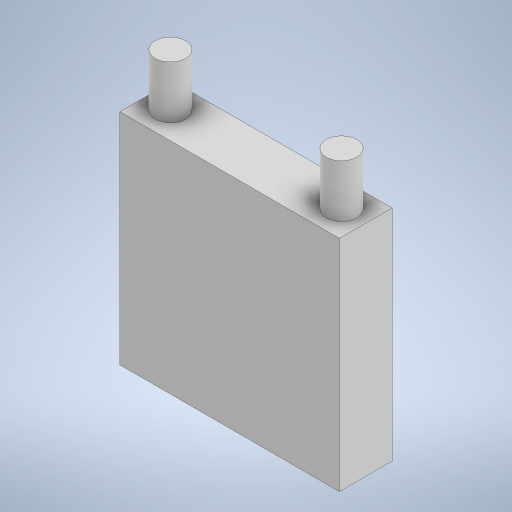
# Autodesk Inventor part: watercoolerpatch
Saved by Autodesk Inventor 2023 (Build 270158000, 158)
## iProperties
Created: 2023-06-13
Part Number: watercoolerpatch
Material: 一般
Document SubType Name: Modeling
Designer: 310611102
Density: 1 g/cm^3
Appearance: 預設
Author: 310611102
Autodesk Inventor part; units mm, degrees
ref_plane "YZ Plane" through (0, 0, 0) normal (1, 0, 0) x (0, 1, 0)
ref_plane "XZ Plane" through (0, 0, 0) normal (0, 1, 0) x (-1, 0, 0)
ref_plane "XY Plane" through (0, 0, 0) normal (0, 0, 1) x (1, 0, 0)
sketch "Sketch1" plane through (0, 0, 0) normal (0, 0, 1) x (1, 0, 0)
  line L0 (-12.5, 12.5) -> (12.5, 12.5)
  line L1 (12.5, 12.5) -> (12.5, -12.5)
  line L2 (12.5, -12.5) -> (-12.5, -12.5)
  line L3 (-12.5, -12.5) -> (-12.5, 12.5)
  line L4 (-12.5, 12.5) -> (12.5, -12.5) construction
  line L5 (12.5, 12.5) -> (-12.5, -12.5) construction
  point P0 (0, 0)
  dimension "d0" = 25
  dimension "d1" = 25
  constraints: 12 end point, 2 midpoint, 2 parallel, 1 horizontal, 1 perpendicular
  measures "d0" distance of L0.start L0.end
  measures "d1" distance of L0.end L1.end
extrude "Extrusion1" add sketch "Sketch1" along normal blind 6
sketch "Sketch2" plane through (-12.5, 12.5, 0) normal (0, 1, 0) x (1, 0, 0)
  circle A0 centre (2.75, -3) radius 1.75
  circle A1 centre (22.25, -3) radius 1.75
  line L0 (25, -6) -> (0, -6) projected
  line L1 (0, 0) -> (0, -6) projected
  line L2 (25, 0) -> (25, -6) projected
  point P0 (12.5, 0)
  dimension "d4" = 3
  dimension "d5" = 3.5
  dimension "d6" = 3.5
  dimension "d7" = 2.75
  dimension "d8" = 2.75
  constraints: 2 centre point, 1 horizontal alignment
  measures "d4" distance from line of A0.centre L0
  measures "d5" diameter of A0
  measures "d6" diameter of A1
  measures "d7" distance from line of L1 A0.centre
  measures "d8" distance from line of L2 A1.centre
extrude "Extrusion2" add sketch "Sketch2" along normal blind 6
body "Solid1"
